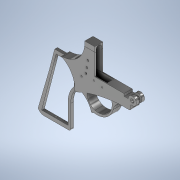
# Autodesk Inventor part: Part19
Saved by Autodesk Inventor 2021 (Build 250183000, 183)
## iProperties
Created: 2020-11-06
Part Number: Part19
Material: Nickel-Copper Alloy 400
Document SubType Name: Modeling
Designer: pedro
Density: 8.83 g/cm^3
Appearance: Chrome - Polished Black
Author: pedro
Autodesk Inventor part; units mm, degrees
ref_plane "YZ Plane" through (0, 0, 0) normal (1, 0, 0) x (0, 1, 0)
ref_plane "XZ Plane" through (0, 0, 0) normal (0, 1, 0) x (-1, 0, 0)
sketch "Sketch1" plane through (0, 0, 0) normal (0, 0, 1) x (1, 0, 0)
  line L0 (0, 0) -> (45, 0) construction
  line L1 (45, 0) -> (45, 69) construction
  line L2 (45, 69) -> (0, 69) construction
  line L3 (0, 69) -> (0, 0) construction
  line L4 (0, 44) -> (45, 44) construction
  line L5 (8.2, 0) -> (37.47, 0) construction
  line L6 (37.47, 0) -> (37.47, 26.36)
  arc A0 (45, 43.997) -> (37.47, 26.36) centre (61.89, 26.36) ccw
  arc A1 (45, 44) -> (35.1527, 65.8492) centre (19.1429, 45.49) ccw
  arc A2 (45, 43.997) -> (30.0099, 69.0002) centre (19.1429, 45.49) ccw
  line L7 (30.0099, 69.0002) -> (20.0099, 69)
  arc A3 (1.8899, 4.0939) -> (8.2, 0) centre (8.2, 6.91) ccw
  line L8 (20.0099, 69) -> (13.9517, 45.6739)
  line L9 (13.9517, 45.6739) -> (1.8899, 4.0939)
  line L10 (0, 69) -> (0, 89.9702) construction
  line L11 (0, 89.9702) -> (45, 89.9702) construction
  line L12 (45, 89.9702) -> (45, 69) construction
  line L13 (30.0099, 69.0002) -> (30.0099, 89.9702) construction
  arc A4 (30.0099, 69.0002) -> (45, 89.9666) centre (20.0214, 91.9834) ccw
  line L14 (45, 43.997) -> (45.4781, 43.6711)
  line L15 (47.7018, 43.6513) -> (48.2287, 43.997)
  arc A5 (45.4781, 43.6711) -> (47.7018, 43.6513) centre (46.6047, 45.3236) ccw
  arc A6 (96.5647, 55.2622) -> (48.2287, 43.997) centre (101.5171, -75.3185) ccw
  line L16 (96.5647, 55.2622) -> (104.4694, 55.2622)
  line L17 (106.4694, 57.2622) -> (106.4694, 61.003)
  arc A7 (104.4694, 55.2622) -> (106.4694, 57.2622) centre (104.4694, 57.2622) ccw
  circle A8 centre (107.8788, 65.2766) radius 4.5
  line L18 (99.9292, 60.7498) -> (99, 60.7498)
  line L19 (99, 60.7498) -> (99, 65.2751)
  line L20 (99, 65.2751) -> (103.3788, 65.2751)
  line L21 (99.9292, 60.7498) -> (106.4694, 60.7498)
  line L22 (99, 60.7498) -> (53, 60.7498)
  line L23 (53, 60.7498) -> (53, 89.965)
  line L24 (53, 89.965) -> (55, 89.965)
  line L25 (55, 90.965) -> (45, 90.965)
  line L26 (45, 90.965) -> (45, 89.9666)
  line L27 (45, 90.965) -> (45, 91.965)
  line L28 (45, 91.965) -> (55, 91.965)
  line L29 (8.2, 0) -> (37.47, 0)
  line L30 (55, 89.965) -> (55, 96.108)
  line L31 (45, 91.965) -> (45, 96.108)
  line L32 (45, 96.108) -> (55, 96.108)
  point P0 (48.9889, 94.5605)
  dimension "d1" = 69
  dimension "d2" = 45
  dimension "d3" = 44
  dimension "d4" = 29.27
  dimension "d5" = 8.2
  dimension "d6" = 26.36
  dimension "d7" = 24.42
  dimension "d8" = 1.49
  dimension "d9" = 25.9
  dimension "d10" = 25.9002
  dimension "d11" = 10
  dimension "d12" = 6.91
  dimension "d13" = 104.56
  dimension "d14" = 24.1
  dimension "d15" = 41.58
  dimension "d16" = 20.97
  dimension "d17" = 25.0599
  dimension "d18" = 20.9666
  dimension "d19" = 14.9901
  dimension "d20" = 2
  dimension "d21" = 130.6746
  dimension "d22" = 2
  dimension "d23" = 9
  dimension "d24" = 1
  dimension "d25" = 1
  dimension "d26" = 2
  dimension "d27" = 10
  dimension "d28" = 46
  dimension "d29" = 7.9047
  dimension "d30" = 3.7408
  dimension "d121" = 6.143
  constraints: 66 end point, 18 point on circle, 13 perpendicular, 10 point on line, 9 centre point, 5 horizontal, 5 tangent, 5 vertical, 2 coincident, 2 collinear
  measures "d1" distance of L0.end L1.end
  measures "d2" distance of L1.end L2.end
  measures "d3" distance of L0.end L4.end
  measures "d4" distance of L5.start L5.end
  measures "d5" distance of L0.start L5.start
  measures "d6" distance of L5.end L6.end
  measures "d7" radius of A0
  measures "d8" distance from line of L4 point (19.143, 45.49)
  measures "d9" radius of A1
  measures "d10" radius of A2
  measures "d11" distance of L7.start L7.end
  measures "d12" radius of A3
  measures "d13" angle of L8 L7
  measures "d14" distance of L7.end L8.end
  measures "d15" vertical distance of L9.end L8.end
  measures "d16" distance of L7.start L13.end
  measures "d17" radius of A4
  measures "d18" distance of L1.end L26.end
  measures "d19" distance of L26.end L13.end
  measures "d20" radius of A5
  measures "d21" radius of A6
  measures "d22" radius of A7
  measures "d23" diameter of A8
  measures "d24" distance of L24.end L25.start
  measures "d25" distance of L28.end L25.start
  measures "d26" distance of L23.end L24.end
  measures "d27" distance of L27.end L28.end
  measures "d28" distance of L18.end L22.end
  measures "d29" distance of L16.start L16.end
  measures "d30" distance of L17.start L17.end
  measures "d121" distance of L24.end L30.end
extrude "Extrusion1" add sketch "Sketch1" along normal mid plane 8.98 contours L29 A3 L9 L8 L7 A2 A1 A0 L6
extrude "Extrusion2" add sketch "Sketch1" along normal mid plane 8.98 contours A2 A1 A4 L26 L25 L30 L24 L23 L22 L18 L21 L17 A7 L16 A6 L15 A5 L14
extrude "Extrusion4" add sketch "Sketch1" along normal mid plane 9 contours L27 L28 L30 L25 | L31 L32 L30 L28
extrude "Extrusion6" add sketch "Sketch1" along normal mid plane 8.98 contours L21 L18 L19 L20 A8 L17
sketch "Sketch3" plane through (0, 0, 4.49) normal (0, 0, 1) x (1, 0, 0)
  line L0 (13.9517, 45.6739) -> (1.8899, 4.0939) construction
  line L1 (1.8899, 4.0939) -> (37.47, 4.0939) construction
  line L2 (37.47, 0) -> (37.47, 26.36) construction
  arc A0 (41.2682, 44.2125) -> (29.4161, 65.1273) centre (19.1429, 45.49) ccw
  arc A1 (45, 43.997) -> (37.47, 26.36) centre (61.89, 26.36) ccw construction
  arc A2 (41.2682, 44.2125) -> (34.6142, 26.36) centre (61.89, 26.36) ccw
  line L3 (34.6142, 26.36) -> (34.6142, 4.0939)
  line L4 (30.0099, 69.0002) -> (20.0099, 69) construction
  line L5 (21.596, 69) -> (21.596, 4.0939) construction
  line L6 (29.4161, 65.1273) -> (21.596, 65.1273)
  line L7 (21.596, 65.1273) -> (5.7435, 4.0939)
  line L8 (5.7435, 4.0939) -> (34.6142, 4.0939)
  point P0 (0, 0)
  dimension "d49" = 104.56
  constraints: 12 end point, 6 point on line, 4 point on circle, 3 perpendicular, 2 centre point, 2 coincident, 2 horizontal
  measures "d49" angle of L6 L7
extrude "Extrusion8" cut sketch "Sketch3" against normal through all
extrude "Extrusion9" add sketch "Sketch1" along normal mid plane 15 contours A8
extrude "Extrusion10" cut sketch "Sketch1" along normal mid plane 15 contours A8
sketch "Sketch4" plane through (53, 60.7498, 4.49) normal (1, 0, 0) x (0, 0, -1)
  point P0 (4.49, -60.7498)
extrude "Extrusion17" add sketch "Sketch1" along normal mid plane 8.98 contours A8
sketch "Sketch6" plane through (0, 0, 4.49) normal (0, 0, 1) x (1, 0, 0)
  arc A0 (106.4694, 61.003) -> (103.3788, 65.2751) centre (107.8788, 65.2766) ccw projected
  circle A1 centre (107.8788, 65.2766) radius 2
  point P0 (0, 0)
  dimension "d78" = 4
  constraints: 1 centre point, 1 coincident
  measures "d78" diameter of A1
extrude "Extrusion18" cut sketch "Sketch6" against normal through all
extrude "Extrusion19" cut sketch "Sketch1" along normal mid plane 8 contours A8
fillet "Arredondamento1" radius 2 1 edges at (37.47, 0, 0)
sketch "Esboço7" plane through (0, 0, 4) normal (0, 0, -1) x (-1, 0, 0)
  circle A0 centre (-107.8788, 65.2766) radius 2 projected
  circle A1 centre (-107.8788, 65.2766) radius 2
  circle A2 centre (-107.8788, 65.2766) radius 4.5
  point P0 (0, 0)
  constraints: 2 centre point, 2 coincident
extrude "Extrusão20" add sketch "Esboço7" along normal blind 2.49
sketch "Esboço8" plane through (0, 0, -4) normal (0, 0, 1) x (1, 0, 0)
  circle A0 centre (107.8823, 65.2751) radius 2.0038
  circle A1 centre (107.8788, 65.2766) radius 2 projected
  circle A2 centre (107.8788, 65.2766) radius 4.5
  point P0 (0, 0)
  point P1 (105.9613, 65.845)
  point P2 (106.1443, 66.2722)
  constraints: 2 centre point, 1 coincident
extrude "Extrusão21" add sketch "Esboço8" along normal blind 2.49 contours A2
sketch "Esboço9" plane through (0, 0, 4.49) normal (0, 0, 1) x (1, 0, 0)
  line L0 (20.0099, 69) -> (13.9517, 45.6739) projected
  arc A0 (35.47, 0) -> (37.47, 2) centre (35.47, 2) ccw projected
  line L1 (37.47, 2) -> (37.47, 26.36) projected
  arc A1 (45, 43.997) -> (37.47, 26.36) centre (61.89, 26.36) ccw projected
  line L2 (45, 43.997) -> (45.4781, 43.6711) projected
  arc A2 (45.4781, 43.6711) -> (47.7018, 43.6513) centre (46.6047, 45.3236) ccw projected
  line L3 (47.7018, 43.6513) -> (48.2287, 43.997) projected
  arc A3 (96.5647, 55.2622) -> (48.2287, 43.997) centre (101.5171, -75.3185) ccw projected
  line L4 (96.5647, 55.2622) -> (104.4694, 55.2622) projected
  arc A4 (104.4694, 55.2622) -> (106.4694, 57.2622) centre (104.4694, 57.2622) ccw projected
  line L5 (106.4694, 57.2622) -> (106.4694, 61.003) projected
  arc A5 (106.4694, 61.003) -> (103.3788, 65.2751) centre (107.8788, 65.2766) ccw projected
  line L6 (103.3788, 65.2751) -> (99, 65.2751) projected
  line L7 (99, 65.2751) -> (99, 60.7498) projected
  line L8 (99, 60.7498) -> (53, 60.7498) projected
  line L9 (53, 60.7498) -> (53, 89.965) projected
  line L10 (53, 89.965) -> (55, 89.965) projected
  line L11 (45, 90.965) -> (45, 89.9666) projected
  arc A6 (30.0099, 69.0002) -> (45, 89.9666) centre (20.0214, 91.9834) ccw projected
  line L12 (30.0099, 69.0002) -> (20.0099, 69) projected
  line L13 (20.0099, 69) -> (13.9517, 45.6739) projected
  line L14 (13.9517, 45.6739) -> (1.8899, 4.0939) projected
  arc A7 (1.8899, 4.0939) -> (8.2, 0) centre (8.2, 6.91) ccw projected
  line L15 (8.2, 0) -> (35.47, 0) projected
  circle A8 centre (107.8788, 65.2766) radius 2 projected
  line L16 (5.7435, 4.0939) -> (21.596, 65.1273) projected
  line L17 (21.596, 65.1273) -> (29.4161, 65.1273) projected
  arc A9 (41.2682, 44.2125) -> (29.4161, 65.1273) centre (19.1429, 45.49) ccw projected
  arc A10 (41.2682, 44.2125) -> (34.6142, 26.36) centre (61.89, 26.36) ccw projected
  line L18 (34.6142, 26.36) -> (34.6142, 4.0939) projected
  line L19 (34.6142, 4.0939) -> (5.7435, 4.0939) projected
  arc A11 (45, 43.997) -> (30.0099, 69.0002) centre (19.1431, 45.4901) ccw
  line L20 (55, 89.965) -> (55, 90.965) projected
  line L21 (55, 90.965) -> (45, 90.965) projected
  point P0 (0, 0)
  dimension "d88" = 25.9
  constraints: 2 point on circle, 1 centre point
  measures "d88" radius of A11
extrude "Extrusão22" cut sketch "Esboço9" against normal blind 3 contours L12 A11 A1 L1 A0 L15 A7 L14 L0
mirror "Espelhamento1" about plane through (0, 0, 0) normal (0, 0, 1) of "Extrusão22"
sketch "Esboço10" plane through (53, 60.7498, 4.49) normal (0, 1, 0) x (1, 0, 0)
  circle A0 centre (3, 4.49) radius 1
  circle A1 centre (36.88, 4.49) radius 1
  line L0 (0, 8.98) -> (0, 0) projected
  line L1 (46, 0) -> (0, 0) projected
  point P0 (-53, 4.49)
  dimension "d91" = 2
  dimension "d92" = 2
  dimension "d93" = 33.88
  dimension "d94" = 3
  dimension "d96" = 4.49
  dimension "d97" = 4.49
  constraints: 2 centre point
  measures "d91" diameter of A1
  measures "d92" diameter of A0
  measures "d93" distance of A0.centre A1.centre
  measures "d94" distance from line of L0 A0.centre
  measures "d96" distance from line of L1 A0.centre
  measures "d97" distance from line of L1 A1.centre
sketch "Esboço11" plane through (53, 60.7498, 4.49) normal (1, 0, 0) x (0, 0, -1)
  line L0 (0, -16.7528) -> (0, 8.2504) projected
  line L1 (0, 0) -> (8.98, 0)
  line L2 (8.98, 29.2152) -> (0, 29.2152) projected
  line L3 (0, 0) -> (0, 29.2152) projected
  line L4 (8.98, 0) -> (0, 0) projected
  line L5 (8.98, 29.2152) -> (8.98, 0) projected
  point P0 (4.49, -60.7498)
  constraints: 2 end point, 1 horizontal, 1 point on line
extrude "Extrusão24" add sketch "Esboço11" along normal blind 12
sketch "Esboço14" plane through (0, 0, -4.49) normal (0, 0, -1) x (-1, 0, 0)
  circle A0 centre (-102.5764, 60.2991) radius 1
  circle A1 centre (-107.8788, 65.2766) radius 2 projected
  line L0 (-99, 65.2751) -> (-103.3788, 65.2751) projected
  line L1 (-106.4694, 61.003) -> (-106.4694, 57.2622) projected
  point P0 (0, 0)
  dimension "d114" = 2
  dimension "d116" = 4.976
  dimension "d117" = 3.893
  constraints: 1 centre point
  measures "d114" diameter of A0
  measures "d116" distance from line of A0.centre L0
  measures "d117" distance from line of L1 A0.centre
extrude "Extrusão27" cut sketch "Esboço14" against normal blind 4 contours A0
sketch "Sketch16" plane through (65, 60.7498, 4.49) normal (1, 0, 0) x (0, 0, -1)
  line L0 (8.98, 29.2152) -> (0, 29.2152) projected
  line L1 (0, 29.2152) -> (0, 0) projected
  line L2 (8.98, 0) -> (0, 0) projected
  line L3 (8.98, 0) -> (8.98, 29.2152) projected
  point P0 (4.49, -60.7498)
extrude "Extrusion29" add sketch "Sketch16" along normal blind 1.8
sketch "Sketch17" plane through (55, 90.965, 4.5) normal (1, 0, 0) x (0, 0, -1)
  line L0 (9, 5.143) -> (0, 5.143) projected
  line L1 (0, 0) -> (0, 5.143) projected
  line L2 (0.01, 0) -> (0, 0) projected
  line L3 (0.01, -1) -> (0.01, 0) projected
  line L4 (0.01, -1) -> (8.99, -1) projected
  line L5 (8.99, 0) -> (8.99, -1) projected
  line L6 (9, 0) -> (8.99, 0) projected
  line L7 (9, 5.143) -> (9, 0) projected
  point P0 (4.5, -90.965)
extrude "Extrusion30" add sketch "Sketch17" along normal blind 11.7965
sketch "Sketch18" plane through (99, 60.7498, 4.49) normal (0, 1, 0) x (1, 0, 0)
  line L0 (-32.2, 8.98) -> (-32.2, 0) projected
  line L1 (0, 0) -> (-32.2, 0) projected
  line L2 (0, 0) -> (0, 8.98) projected
  line L3 (-32.2, 8.98) -> (0, 8.98) projected
  point P0 (-99, 4.49)
extrude "Extrusion31" add sketch "Sketch18" along normal blind 7
sketch "Sketch23" plane through (0, 0, 4.49) normal (0, 0, 1) x (1, 0, 0)
  line L0 (106.4694, 57.2622) -> (106.4694, 61.003) projected
  arc A0 (106.4694, 61.003) -> (103.3788, 65.2751) centre (107.8788, 65.2766) ccw projected
  line L1 (103.3788, 65.2751) -> (99, 65.2751) projected
  line L2 (66.8, 89.965) -> (66.8, 67.7498) projected
  line L3 (66.7965, 90.965) -> (66.7965, 89.965) projected
  line L4 (66.7965, 90.965) -> (45, 90.965) projected
  line L5 (45, 90.965) -> (45, 89.9666) projected
  arc A1 (30.0099, 69.0002) -> (45, 89.9666) centre (20.0214, 91.9834) ccw projected
  arc A2 (45, 43.997) -> (30.0099, 69.0002) centre (19.1431, 45.4901) ccw projected
  line L6 (45, 43.997) -> (45.4781, 43.6711) projected
  arc A3 (45.4781, 43.6711) -> (47.7018, 43.6513) centre (46.6047, 45.3236) ccw projected
  line L7 (47.7018, 43.6513) -> (48.2287, 43.997) projected
  arc A4 (96.5647, 55.2622) -> (48.2287, 43.997) centre (101.5171, -75.3185) ccw projected
  line L8 (96.5647, 55.2622) -> (104.4694, 55.2622) projected
  arc A5 (104.4694, 55.2622) -> (106.4694, 57.2622) centre (104.4694, 57.2622) ccw projected
  circle A6 centre (107.8788, 65.2766) radius 2 projected
  line L9 (45, 96.108) -> (45, 90.965) projected
  line L10 (45, 96.108) -> (66.7965, 96.108)
  line L11 (30.0099, 69.0002) -> (57.7131, 69.0002)
  arc A7 (45, 43.997) -> (30.0099, 69.0002) centre (19.1431, 45.4901) ccw projected
  line L12 (45, 96.108) -> (66.7965, 96.108) projected
  arc A8 (30.0099, 69.0002) -> (55.8983, 96.108) centre (30.8589, 94.1051) ccw
  line L13 (99, 65.2751) -> (99, 67.7498) projected
  line L14 (66.8, 67.7498) -> (99, 67.7498) projected
  line L15 (66.7965, 89.965) -> (66.8, 89.965) projected
  point P0 (0, 0)
  point P1 (31.7079, 69.0002)
  point P2 (55.8983, 96.108)
  constraints: 4 end point, 2 horizontal, 2 point on circle, 1 centre point, 1 midpoint
extrude "Extrusion34" cut sketch "Sketch23" against normal mid plane 20 contours A1 L5 L4 A8 L11 | L4 L9 L10 A8
sketch "Sketch22" plane through (66.8, 60.7498, 4.49) normal (1, 0, 0) x (0, 0, -1)
  line L0 (8.98, 7) -> (8.98, 29.2152) projected
  line L1 (0, 29.2152) -> (0, 7) projected
  line L2 (1.49, 6.9153) -> (7.49, 6.9234)
  line L3 (1.49, 31.9153) -> (1.49, 6.9153)
  line L4 (5.98, 8.2504) -> (3, 8.2504) projected
  line L5 (0, 8.2504) -> (8.98, 8.2504)
  line L6 (0, 7) -> (8.98, 7) projected
  line L7 (7.49, 6.9234) -> (7.49, 8.2504)
  line L8 (7.49, 8.2504) -> (7.49, 31.9153)
  arc A0 (7.49, 31.9153) -> (1.49, 31.9153) centre (4.49, 31.9153) ccw
  line L9 (8.98, 29.2152) -> (0, 29.2152) projected
  point P0 (4.49, -60.7498)
  point P1 (1.49, 8.2504)
  dimension "d143" = 6
  dimension "d164" = 1.49
  dimension "d165" = 1.49
  constraints: 10 end point, 3 point on line, 2 point on circle, 2 tangent, 1 centre point, 1 perpendicular, 1 vertical
  measures "d143" distance of L2.start L2.end
  measures "d164" distance between parallel lines of L3 L1
  measures "d165" distance between parallel lines of L0 L8
extrude "Extrusion33" cut sketch "Sketch22" against normal blind 23 contours L7 L2 L3 L6 | L6 L3 L5 L4 L7 | L5 L4 L3 L9 L8 | L9 L3 A0 L8
chamfer "Chamfer2" distance 0.5 angle 45 2 edges at (30.0099, 69.0002, -2.99) (30.0099, 69.0002, 2.99)
sketch "Esboço26" plane through (99, 67.7498, 4.49) normal (0, 1, 0) x (1, 0, 0)
  line L0 (-32.2, 1.49) -> (-32.2, 7.49) projected
  line L1 (-32.2, 7.49) -> (-32.2, 8.98) projected
  line L2 (-32.2, 0) -> (0, 0) projected
  line L3 (0, 8.98) -> (-32.2, 8.98) projected
  line L4 (-32.2, 0) -> (-32.2, 1.49) projected
  line L5 (-34.9559, 0.9925) -> (-23.46, 0.9925)
  line L6 (-23.46, 7.9925) -> (-34.9559, 7.9925)
  line L7 (-23.46, 7.9925) -> (-19.5, 7.9925)
  line L8 (-19.5, 7.9925) -> (-19.5, 0.9925)
  line L9 (-19.5, 0.9925) -> (-23.46, 0.9925)
  line L10 (-34.9559, 0.9925) -> (-37.9592, 0.9925)
  line L11 (-37.9592, 0.9925) -> (-37.9592, 7.9925)
  line L12 (-32.2, 7.49) -> (-55.2, 7.49) projected
  line L13 (-37.9592, 7.9925) -> (-32.2, 7.9925)
  point P0 (-99, 4.49)
  point P1 (-32.2, 0.9925)
  point P2 (-29.8, 7.9925)
  dimension "d158" = 8.98
  dimension "d160" = 7
  dimension "d162" = 0.9875
  dimension "d163" = 12.7
  constraints: 16 end point, 4 perpendicular, 2 horizontal, 2 point on line, 1 collinear
  measures "d158" distance between parallel lines of L2 L3
  measures "d160" distance between parallel lines of L5 L6
  measures "d162" distance between parallel lines of L3 L6
  measures "d163" distance between parallel lines of L8 L1
extrude "Extrusão37" cut sketch "Esboço26" against normal through all
fillet "Arredondamento3" radius 1 2 edges at (63.9204, 67.7498, -3) (63.9204, 67.7498, 3)
sketch "Esboço29" plane through (61.0408, 48.9293, 3.4975) normal (1, 0, 0) x (0, 0, -1)
  line L0 (0, 18.8205) -> (0, 0) projected
  line L1 (7, 18.8205) -> (7, 0) projected
  line L2 (0, 18.8205) -> (7, 18.8205)
  line L3 (7, 18.8205) -> (7, 3.8205)
  line L4 (7, 3.8205) -> (0, 3.8205)
  line L5 (0, 3.8205) -> (0, 18.8205)
  point P0 (3.4975, -48.9293)
  point P1 (0, 3.8205)
  dimension "d170" = 15
  constraints: 8 end point, 3 perpendicular, 1 horizontal
  measures "d170" distance between parallel lines of L4 L2
extrude "Extrusão39" cut sketch "Esboço29" against normal blind 17
ref_plane "Plano de trabalho4" through (44.0408, 52.7498, 3.4975) normal (0.8660254, 0.5, 0) x (0, 0, 1)
sketch "Esboço30" plane through (44.0408, 52.7498, 3.4975) normal (0.8660254, 0.5, 0) x (0, 0, 1)
  line L0 (0, 4.7392) -> (0, -1.6108) projected
  line L1 (0, 3.1606) -> (-6.9895, 3.1606)
  line L2 (-6.9895, 3.1606) -> (-7, -8.7404)
  line L3 (-7, -4.4904) -> (-7, -12.9904) projected
  line L4 (0, -4.4904) -> (0, -12.9904) projected
  line L5 (0, -8.364) -> (0, 3.817)
  line L6 (-7, -8.7404) -> (0, -8.7404)
  line L7 (0, -8.7404) -> (0, -8.364)
  point P0 (-3.4975, 23.6623)
  point P1 (0, -4.4904)
  constraints: 10 end point, 2 collinear, 2 midpoint, 2 point on line, 1 horizontal
extrude "Extrusão40" cut sketch "Esboço30" against normal mid plane 17
sketch "Esboço31" plane through (8.2, 0, 1.49) normal (0, -1, 0) x (1, 0, 0)
  line L0 (11.8099, 0) -> (11.8099, -2.98) projected
  circle A0 centre (11.8099, -1.49) radius 0.9
  point P0 (-8.2, -1.49)
  dimension "d176" = 1.8
  constraints: 1 centre point, 1 midpoint
  measures "d176" diameter of A0
extrude "Extrusão41" cut sketch "Esboço31" against normal blind 14
sketch "Esboço32" plane through (0, 0, -4.49) normal (0, 0, -1) x (-1, 0, 0)
  circle A0 centre (-59.332, 79.579) radius 1
  line L0 (-55.8983, 96.108) -> (-66.7965, 96.108) projected
  line L1 (-66.8, 67.7498) -> (-66.8, 89.965) projected
  point P0 (0, 0)
  dimension "d179" = 2
  dimension "d180" = 16.529
  dimension "d181" = 7.468
  constraints: 1 centre point
  measures "d179" diameter of A0
  measures "d180" distance from line of A0.centre L0
  measures "d181" distance from line of L1 A0.centre
extrude "Extrusão42" cut sketch "Esboço32" against normal blind 14
sketch "Esboço33" plane through (0, 0, 4.49) normal (0, 0, 1) x (1, 0, 0)
  arc A0 (63.1318, 32.7254) -> (64.573, 32.6074) centre (63.8753, 32.9462) ccw
  line L0 (64.573, 32.6074) -> (65.7995, 33.1581)
  arc A1 (65.7995, 33.1581) -> (87.0962, 46.8053) centre (69.2993, 51.1371) ccw
  arc A2 (63.1318, 32.7254) -> (52.8076, 45.9904) centre (41.0081, 26.1565) ccw
  arc A3 (58.3891, 48.0759) -> (66.9436, 36.0308) centre (70.9284, 47.9211) ccw
  arc A4 (85.4415, 47.1972) -> (85.3705, 54.3533) centre (70.7489, 50.6298) ccw
  arc A5 (92.4951, 55.0323) -> (87.0962, 46.8053) centre (101.3507, 43.3358) ccw
  arc A6 (58.3891, 48.0759) -> (52.8076, 45.9904) centre (101.3247, -75.3436) ccw
  arc A7 (92.4951, 55.0323) -> (85.3705, 54.3533) centre (101.3247, -75.3436) ccw
  arc A8 (66.9436, 36.0308) -> (85.4415, 47.1972) centre (70.7505, 50.629) ccw
  point P0 (0, 0)
  constraints: 18 point on circle, 9 centre point, 2 end point, 2 tangent
extrude "Extrusão43" add sketch "Esboço33" against normal up to surface (8.98 mm away)
sketch "Esboço34" plane through (79.5, 53.4879, 3.4975) normal (0, 0, -1) x (-1, 0, 0)
  line L0 (12.7, 14.2619) -> (12.7, 15.1264) projected
  line L1 (12.7, 14.2619) -> (10.7, 14.2619) construction
  line L2 (-19.5, 14.2619) -> (12.7, 14.2619) projected
  line L3 (10.7, 14.2619) -> (4.546, 8.2714) construction
  circle A0 centre (4.546, 8.2714) radius 0.75
  point P0 (79.5, -53.4879)
  dimension "d186" = 2
  dimension "d188" = 1.5
  constraints: 4 end point, 1 centre point, 1 coincident, 1 point on line
  measures "d186" distance of L0.start L1.end
  measures "d188" diameter of A0
extrude "Extrusão44" cut sketch "Esboço34" against normal up to surface (0.9925 mm away)
sketch "Esboço35" plane through (0, 0, 4.49) normal (0, 0, 1) x (1, 0, 0)
  circle A0 centre (65.8788, 63.6563) radius 0.75
  point P0 (0, 0)
  dimension "d191" = 1.5
  constraints: 1 centre point
  measures "d191" diameter of A0
extrude "Extrusão45" cut sketch "Esboço35" against normal up to surface (0.9925 mm away)
sketch "Esboço36" plane through (0, 0, 4.49) normal (0, 0, 1) x (1, 0, 0)
  circle A0 centre (57.1985, 66.0664) radius 1
  point P0 (0, 0)
  dimension "d194" = 2
  constraints: 1 centre point
  measures "d194" diameter of A0
extrude "Extrusão47" cut sketch "Esboço36" against normal up to surface (1.49 mm away)
sketch "Esboço37" plane through (0, 0, 4.49) normal (0, 0, 1) x (1, 0, 0)
  circle A0 centre (58.2353, 72.1644) radius 1
  point P0 (0, 0)
  dimension "d199" = 2
  constraints: 1 centre point
  measures "d199" diameter of A0
extrude "Extrusão48" cut sketch "Esboço37" against normal up to surface (1.49 mm away)
sketch "Esboço38" plane through (0, 0, 4.49) normal (0, 0, 1) x (1, 0, 0)
  circle A0 centre (52.4566, 61.0058) radius 0.75
  point P0 (0, 0)
  dimension "d202" = 1.5
  constraints: 1 centre point
  measures "d202" diameter of A0
extrude "Extrusão49" cut sketch "Esboço38" against normal up to surface (0.9925 mm away)
body "Solid1"
